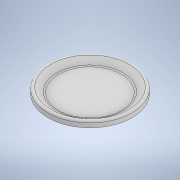
# Autodesk Inventor part: 77. Заглушка
Saved by Autodesk Inventor 2021 (Build 250183000, 183)
## iProperties
Created: 2021-03-15
Part Number: 77. Заглушка
Material: Типовые
Document SubType Name: Modeling
Designer: Данил
Density: 1 g/cm^3
Appearance: По умолчанию
Author: Данил
Autodesk Inventor part; units mm, degrees
ref_plane "YZ Plane" through (0, 0, 0) normal (1, 0, 0) x (0, 1, 0)
ref_plane "XZ Plane" through (0, 0, 0) normal (0, 1, 0) x (-1, 0, 0)
ref_plane "XY Plane" through (0, 0, 0) normal (0, 0, 1) x (1, 0, 0)
sketch "Эскиз1" plane through (0, 0, 0) normal (0, 0, 1) x (1, 0, 0)
  line L0 (0, 3.25) -> (0, -3.25)
  line L1 (0, -2.25) -> (33.5687, -2.25)
  line L2 (35.2894, -1.7075) -> (41.8528, 2.8883)
  line L3 (45, 1.25) -> (45, -3.25)
  arc A0 (33.5687, -2.25) -> (35.2894, -1.7075) centre (33.5687, 0.75) ccw
  arc A1 (45, 1.25) -> (41.8528, 2.8883) centre (43, 1.25) ccw
  line L4 (0, 3.25) -> (45, 3.25) construction
  line L5 (0, -3.25) -> (33.2828, -3.25)
  line L6 (35.0035, -2.7075) -> (40.8528, 1.3883)
  line L7 (44, -0.25) -> (44, -3.25)
  arc A2 (33.2828, -3.25) -> (35.0035, -2.7075) centre (33.2828, -0.25) ccw
  arc A3 (44, -0.25) -> (40.8528, 1.3883) centre (42, -0.25) ccw
  line L8 (44, -3.25) -> (45, -3.25)
  point P0 (0, 0)
  point P1 (0, 0)
  dimension "d0" = 6.5
  dimension "d1" = 1
  dimension "d2" = 3
  dimension "d3" = 55
  dimension "d4" = 90
  dimension "d5" = 2
  dimension "d6" = 55
  dimension "d7" = 3
  dimension "d8" = 2
  dimension "d9" = 1
  constraints: 18 end point, 9 tangent, 8 point on circle, 4 centre point, 4 horizontal, 3 horizontal alignment, 2 point on line, 2 vertical, 1 coincident, 1 midpoint, 1 perpendicular, 1 vertical alignment
  measures "d0" distance of L0.start L0.end
  measures "d1" distance from line of L0.end L1
  measures "d2" radius of A0
  measures "d3" angle of L3 L2
  measures "d4" diameter of L3 L0
  measures "d5" radius of A1
  measures "d6" angle of L7 L6
  measures "d7" radius of A2
  measures "d8" radius of A3
  measures "d9" distance between parallel lines of L3 L7
revolve "Вращение1" add sketch "Эскиз1" angle 360 about axis through (0, 3.25, 0) along (0, -1, 0)
